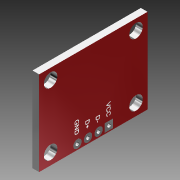
# Autodesk Inventor part: SparkFun USB Type A Female Breakout - doska
Saved by Autodesk Inventor 2013 SP2 (Build 170200200, 200)
## iProperties
Created: 2018-05-07
Part Number: SparkFun USB Type A Female Breakout - doska
Material: ABS plast
Document SubType Name: Modelování
Designer: PCC
Density: 1.06 g/cm^3
Author: PCC
Autodesk Inventor part; units mm, degrees
ref_plane "YZ Plane" through (0, 0, 0) normal (1, 0, 0) x (0, 1, 0)
ref_plane "XZ Plane" through (0, 0, 0) normal (0, 1, 0) x (-1, 0, 0)
ref_plane "XY Plane" through (0, 0, 0) normal (0, 0, 1) x (1, 0, 0)
sketch "Náčrt1" plane through (0, 0, 0) normal (1, 0, 0) x (0, 1, 0)
  line L0 (0, 0) -> (26, 0)
  line L1 (26, 0) -> (26, 20.3)
  line L2 (26, 20.3) -> (0, 20.3)
  line L3 (0, 20.3) -> (0, 0)
  dimension "d0" = 26
  dimension "d1" = 20.3
  constraints: 8 end point, 2 parallel, 1 horizontal, 1 perpendicular
  measures "d0" distance of L0.start L0.end
  measures "d1" distance of L2.end L0.start
extrude "Vysunutí1" add sketch "Náčrt1" along normal blind 1.6
sketch "Náčrt2" plane through (1.6, 0, 0) normal (1, 0, 0) x (0, 0, -1)
  line L0 (0, 0) -> (0, 26) projected
  line L1 (-20.3, 0) -> (0, 0) projected
  circle A0 centre (-2.75, 23.25) radius 1.625
  circle A1 centre (-2.75, 2.75) radius 1.625
  circle A2 centre (-1.27, 16.81) radius 0.45
  circle A3 centre (-1.27, 14.27) radius 0.45
  circle A4 centre (-1.27, 11.73) radius 0.45
  circle A5 centre (-1.27, 9.19) radius 0.45
  circle A6 centre (-17.75, 23.25) radius 1.625
  circle A7 centre (-17.75, 2.75) radius 1.625
  dimension "d4" = 20.5
  dimension "d6" = 3.25
  dimension "d7" = 2.75
  dimension "d8" = 2.75
  dimension "d9" = 2.75
  dimension "d10" = 0.9
  dimension "d11" = 1.27
  dimension "d12" = 2.54
  dimension "d13" = 2.54
  dimension "d14" = 2.54
  dimension "d15" = 1.27
  dimension "d16" = 1.27
  dimension "d17" = 1.27
  dimension "d18" = 7.62
  dimension "d19" = 6.44
  dimension "d20" = 20.5
  dimension "d21" = 2.75
  dimension "d25" = 15
  dimension "d26" = 15
  constraints: 8 centre point, 6 equal radius
  measures "d4" distance of A1.centre A0.centre
  measures "d6" diameter of A0
  measures "d7" distance from line of A1.centre L1
  measures "d8" distance from line of L0 A0.centre
  measures "d9" distance from line of L0 A1.centre
  measures "d10" diameter of A2
  measures "d11" distance from line of L0 A2.centre
  measures "d12" distance of A3.centre A2.centre
  measures "d13" distance of A3.centre A4.centre
  measures "d14" distance of A4.centre A5.centre
  measures "d15" distance from line of L0 A3.centre
  measures "d16" distance from line of L0 A4.centre
  measures "d17" distance from line of L0 A5.centre
  measures "d18" distance of A5.centre A2.centre
  measures "d19" vertical distance of A0.centre A2.centre
  measures "d20" distance of A7.centre A6.centre
  measures "d21" distance from line of A7.centre L1
  measures "d25" distance of A0.centre A6.centre
  measures "d26" distance of A1.centre A7.centre
extrude "Vysunutí3" cut sketch "Náčrt2" against normal through all
sketch "Náčrt3" plane through (1.6, 0, 0) normal (1, 0, 0) x (0, 0, -1)
  circle A0 centre (-1.27, 11.73) radius 0.45 projected
  circle A1 centre (-1.27, 16.81) radius 0.45 projected
  circle A2 centre (-1.27, 14.27) radius 0.45 projected
  circle A3 centre (-1.27, 9.19) radius 0.45 projected
  line L0 (-2.27, 17.7223) -> (-0.27, 17.7223)
  line L1 (-0.27, 17.7223) -> (-0.27, 15.7223)
  line L2 (-0.27, 15.7223) -> (-2.27, 15.7223)
  line L3 (-2.27, 15.7223) -> (-2.27, 17.7223)
  circle A4 centre (-1.27, 14.27) radius 1
  circle A5 centre (-1.27, 11.73) radius 1
  circle A6 centre (-1.27, 9.19) radius 1
  dimension "d31" = 2
  dimension "d33" = 1
  dimension "d34" = 2
  dimension "d35" = 1.0877
  dimension "d36" = 2
  constraints: 8 end point, 3 centre point, 3 coincident, 2 equal radius, 2 parallel, 1 horizontal, 1 perpendicular
  measures "d31" distance of L0.start L0.end
  measures "d33" distance from line of A1.centre L1
  measures "d34" distance of L2.end L0.start
  measures "d35" distance from line of A1.centre L2
  measures "d36" diameter of A4
extrude "Vysunutí4" add sketch "Náčrt3" along normal blind 0.001
sketch "Náčrt4" plane through (0, 0, 0) normal (-1, 0, 0) x (0, 0, 1)
  circle A0 centre (1.27, 11.73) radius 0.45 projected
  circle A1 centre (1.27, 16.81) radius 0.45 projected
  circle A2 centre (1.27, 14.27) radius 0.45 projected
  circle A3 centre (1.27, 9.19) radius 0.45 projected
  line L0 (2.27, 17.7223) -> (0.27, 17.7223) projected
  line L1 (2.27, 15.7223) -> (2.27, 17.7223) projected
  line L2 (0.27, 15.7223) -> (2.27, 15.7223) projected
  line L3 (0.27, 17.7223) -> (0.27, 15.7223) projected
  circle A4 centre (1.27, 14.27) radius 1 projected
  circle A5 centre (1.27, 11.73) radius 1 projected
  circle A6 centre (1.27, 9.19) radius 1 projected
extrude "Vysunutí5" add sketch "Náčrt4" along normal blind 0.001
sketch "Náčrt5" plane through (1.6, 0, 0) normal (1, 0, 0) x (0, 0, -1)
  line L0 (-12.9507, 18.458) -> (-3.259, 18.458) construction
  line L1 (-3.259, 18.458) -> (-3.259, 7.2075) construction
  line L2 (-3.259, 7.2075) -> (-12.9507, 7.2075) construction
  line L3 (-12.9507, 7.2075) -> (-12.9507, 18.458) construction
  constraints: 2 other
sketch "Náčrt6" plane through (0, 0, 0) normal (-1, 0, 0) x (0, 0, 1)
  line L0 (2.7892, 18.5709) -> (6.1278, 18.5709) construction
  line L1 (6.1278, 18.5709) -> (6.1278, 7.3401) construction
  line L2 (6.1278, 7.3401) -> (2.7892, 7.3401) construction
  line L3 (2.7892, 7.3401) -> (2.7892, 18.5709) construction
  line L4 (9.218, 26) -> (9.218, 0) construction
  line L5 (9.218, 0) -> (6.7421, 0) construction
  line L6 (6.7421, 0) -> (6.7421, 26) construction
  line L7 (6.7421, 26) -> (9.218, 26) construction
  line L8 (18.8, 26) -> (18.8, 0) construction
  line L9 (18.8, 0) -> (16.2512, 0) construction
  line L10 (16.2512, 0) -> (16.2512, 26) construction
  line L11 (16.2512, 26) -> (18.8, 26) construction
  constraints: 6 other
equation "\"d7\" = -0.5 * d4 + 0.5 * d0"
equation "\"d8\" = d7"
equation "\"d9\" = d7"
equation "\"d15\" = d11"
equation "\"d16\" = d11"
equation "\"d17\" = d11"
equation "\"d19\" = -0.5 * d18 + 0.5 * d4"
equation "\"d20\" = d4"
equation "\"d21\" = d7"
equation "\"d26\" = d25"
equation "\"PoloměrOhybu\" = Tloušťka"
equation "\"ŠířkaVýštipu\" = Tloušťka"
equation "\"HloubkaVýštipu\" = 0.5 * Tloušťka"
equation "\"VelikostRohovéhoVýštipu\" = 4 * Tloušťka"
equation "\"MinimálníZbytek\" = 2 * Tloušťka"
equation "\"PřechodovýPoloměr\" = PoloměrOhybu"
equation "\"VelikostJacobihoPoloměru\" = Tloušťka"
equation "\"VelikostMezery\" = Tloušťka"
equation "\"Tloušťka\" = 0.5"
